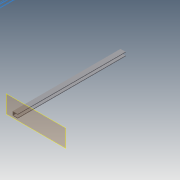
# Autodesk Inventor part: Z-table Rail
Saved by Autodesk Inventor 2014 SP1 (Build 180222100, 222)
## iProperties
Created: 2014-04-10
Part Number: Z-table Rail
Material: Generic
Document SubType Name: Modeling
Designer: tom
Density: 1 g/cm^3
Appearance: Default
Author: tom
Autodesk Inventor part; units mm, degrees
ref_plane "YZ Plane" through (0, 0, 0) normal (1, 0, 0) x (0, 1, 0)
ref_plane "XZ Plane" through (0, 0, 0) normal (0, 1, 0) x (-1, 0, 0)
ref_plane "XY Plane" through (0, 0, 0) normal (0, 0, 1) x (1, 0, 0)
ref_plane "Work Plane1" through (23.8016, -120.6016, 287.3377) normal (0, 0, 1) x (1, 0, 0)
sketch "Sketch1" plane through (23.8016, -120.6016, 287.3377) normal (0, 0, 1) x (1, 0, 0)
  line L0 (-60.325, -11.1235) -> (-60.325, -21.1235)
  line L1 (-60.325, -21.1235) -> (-47.325, -21.1235)
  line L2 (-47.325, -21.1235) -> (-47.325, -19.5235)
  line L3 (-47.325, -19.5235) -> (-58.725, -19.5235)
  line L4 (-58.725, -19.5235) -> (-58.725, -12.7235)
  line L5 (-58.725, -12.7235) -> (-47.3247, -12.7235)
  line L6 (-47.3247, -12.7235) -> (-47.3247, -11.1235)
  line L7 (-47.3247, -11.1235) -> (-60.325, -11.1235)
  point P0 (-23.8016, 120.6016)
  dimension "d0" = 10
  dimension "d1" = 13
  dimension "d2" = 1.6
  dimension "d3" = 1.6
  dimension "d4" = 1.6
  constraints: 16 end point, 4 perpendicular, 3 parallel
  measures "d0" distance of L0.start L0.end
  measures "d1" distance of L0.end L1.end
  measures "d2" distance of L1.end L2.end
  measures "d3" distance of L5.end L6.end
  measures "d4" distance between parallel lines of L0 L4
extrude "Extrusion1" add sketch "Sketch1" against normal blind 286.324
body "Solid1"
